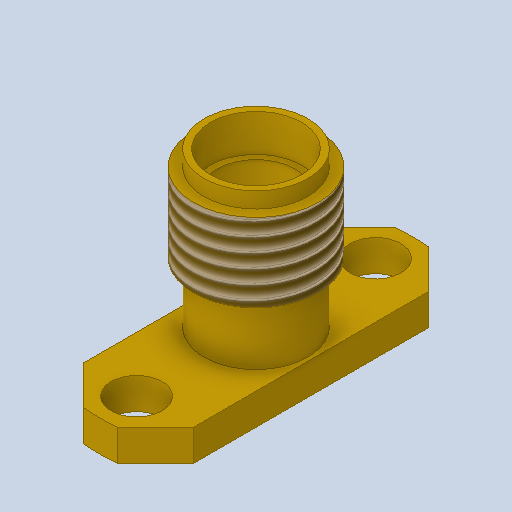
# Autodesk Inventor part: SMA-PanelMount-Ni-AuPlated-Body
Saved by Autodesk Inventor 2026 (Build 300175050, 175E)
## iProperties
Created: 2018-08-15
Part Number: SMA-PanelMount-Ni-AuPlated-Body
Material: Brass
Document SubType Name: Modeling
Designer: schanen
Density: 8.49 g/cm^3
Appearance: Gold
Mass: 4.18807 g
Surface Area: 5.74005 cm^2
Volume: 0.4743 cm^3
Author: schanen
Autodesk Inventor part; units mm, degrees
ref_plane "YZ Plane" through (0, 0, 0) normal (1, 0, 0) x (0, 1, 0)
ref_plane "XZ Plane" through (0, 0, 0) normal (0, 1, 0) x (-1, 0, 0)
ref_plane "XY Plane" through (0, 0, 0) normal (0, 0, 1) x (1, 0, 0)
sketch "Sketch10" plane through (0, 0, 0) normal (0, 0, 1) x (1, 0, 0)
  line L0 (-2, 0) -> (-8, 0)
  line L1 (-8, 0) -> (-8, 1.6)
  line L2 (-8, 1.6) -> (-2.65, 1.6)
  line L3 (-2.65, 1.6) -> (-2.65, 4.7)
  line L4 (-2.65, 4.7) -> (-3.175, 4.7)
  line L5 (-3.175, 4.7) -> (-3.175, 8.7)
  line L6 (-2, 7.6) -> (-2, 0)
  line L7 (-3.175, 8.7) -> (-2.65, 8.7)
  line L8 (-2.65, 8.7) -> (-2.65, 9.5)
  line L9 (-2.65, 9.5) -> (-2.325, 9.5)
  line L10 (0, -1.9) -> (0, 11.4) projected
  line L11 (-2.325, 9.5) -> (-2.325, 7.6)
  line L12 (-2.325, 7.6) -> (-2, 7.6)
  point P0 (0, 0)
  dimension "d39" = 2
  dimension "d41" = 0.8
  dimension "d42" = 4
  dimension "d43" = 2.65
  dimension "d44" = 1.6
  dimension "d45" = 8
  dimension "d46" = 3.175
  dimension "d66" = 2.325
  dimension "d67" = 1.9
  dimension "d68" = 9.5
  constraints: 25 end point, 8 perpendicular, 2 horizontal, 2 vertical alignment, 1 horizontal alignment, 1 vertical
  measures "d39" distance from line of point (0, 0) L6
  measures "d41" distance between parallel lines of L7 L9
  measures "d42" distance of L4.end L5.end
  measures "d43" distance from line of point (0, 0) L3
  measures "d44" distance of L0.end L1.end
  measures "d45" distance from line of point (0, 0) L1
  measures "d46" distance from line of point (0, 0) L5
  measures "d66" distance from line of point (0, 0) L11
  measures "d67" distance of L9.end L11.end
  measures "d68" distance from line of point (0, 0) L9
revolve "Revolution1" add sketch "Sketch10" angle 360 about axis through (0, -10, 0) along (0, 1, 0)
sketch "Sketch11" plane through (0, 0, 0) normal (0, -1, 0) x (1, 0, 0)
  circle A0 centre (0, 0) radius 8 projected
  line L0 (2.825, -7.4846) -> (2.825, 7.4846)
  line L1 (-2.825, -7.4846) -> (-2.825, 7.4846)
  arc A1 (2.825, -7.4846) -> (2.825, 7.4846) centre (0, 0) ccw
  arc A2 (-2.825, 7.4846) -> (-2.825, -7.4846) centre (0, 0) ccw
  dimension "d48" = 5.65
  constraints: 8 point on circle, 4 end point, 2 centre point, 2 coincident, 2 vertical, 1 horizontal alignment
  measures "d48" distance between parallel lines of L0 L1
extrude "Extrusion7" cut sketch "Sketch11" against normal up to surface (1.6 mm away) contours A0 L0 | L1 A0
sketch "Sketch12" plane through (0, 0, 0) normal (0, -1, 0) x (1, 0, 0)
  line L0 (2.825, 7.4846) -> (2.825, -7.4846) projected
  line L1 (2.825, 6) -> (0.8727, 7.9523)
  line L2 (2.825, -6) -> (0.8727, -7.9523)
  arc A0 (-2.825, -7.4846) -> (2.825, -7.4846) centre (0, 0) ccw projected
  arc A1 (2.825, 7.4846) -> (-2.825, 7.4846) centre (0, 0) ccw projected
  line L3 (0, -11.2) -> (0, 11.2) projected
  line L4 (-2.825, 6) -> (-0.8727, 7.9523)
  line L5 (-2.825, -6) -> (-0.8727, -7.9523)
  line L6 (-2.825, 7.4846) -> (-2.825, -7.4846) projected
  dimension "d51" = 12
  dimension "d52" = 6
  dimension "d53" = 45
  dimension "d54" = 45
  constraints: 8 end point, 4 symmetric about line, 2 point on circle, 2 point on line
  measures "d51" distance of L1.start L2.start
  measures "d52" vertical distance of point (0, 0) L1.start
  measures "d53" angle of L1 L0
  measures "d54" angle of L0 L2
extrude "Extrusion8" cut sketch "Sketch12" against normal through all contours L0 L1 A1 | L0 A0 L2 | L4 L6 A1 | A0 L6 L5
sketch "Sketch13" plane through (0, 0, 0) normal (0, -1, 0) x (1, 0, 0)
  point P0 (0, 0)
  point P1 (0, 6.1)
  point P2 (0, -6.1)
  dimension "d57" = 12.2
  dimension "d58" = 6.1
  constraints: 2 vertical alignment
  measures "d57" distance of point (0, 6.1) point (0, -6.1)
  measures "d58" distance of point (0, 0) point (0, 6.1)
hole "Hole3" at (0, 0, 6.1) at (0, 0, -6.1) direction (0, 1, 0) diameter 2.6 end through all
thread "Thread2" size "1/4-36 UNS" class "2A" standard "ANSI Unified Screw Threads" length 9
equation "\"d52\" = 0.5 * d51"
equation "\"d54\" = d53"
equation "\"d58\" = 0.5 * d57"
body "Solid2"
